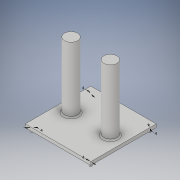
# Autodesk Inventor part: MainStage
Saved by Autodesk Inventor 2019 (Build 230136000, 136)
## iProperties
Created: 2021-06-23
Part Number: MainStage
Material: Generic
Document SubType Name: Modeling
Designer: 91742
Density: 1 g/cm^3
Appearance: Default
Author: 91742
Autodesk Inventor part; units mm, degrees
ref_plane "YZ Plane" through (0, 0, 0) normal (1, 0, 0) x (0, 1, 0)
ref_plane "XZ Plane" through (0, 0, 0) normal (0, 1, 0) x (-1, 0, 0)
ref_plane "XY Plane" through (0, 0, 0) normal (0, 0, 1) x (1, 0, 0)
sketch "Sketch1" plane through (0, 0, 0) normal (0, 1, 0) x (-1, 0, 0)
  line L0 (50, 50) -> (-50, 50)
  line L1 (-50, 50) -> (-50, -50)
  line L2 (-50, -50) -> (50, -50)
  line L3 (50, -50) -> (50, 50)
  line L4 (50, 50) -> (-50, -50) construction
  line L5 (-50, 50) -> (50, -50) construction
  line L6 (-45, 45) -> (45, -45) construction
  line L7 (45, 45) -> (-45, -45) construction
  circle A0 centre (45, -45) radius 2
  circle A1 centre (-45, -45) radius 2
  circle A2 centre (-45, 45) radius 2
  circle A3 centre (45, 45) radius 2
  point P0 (0, 0)
  dimension "d0" = 100
  dimension "d1" = 100
  dimension "d8" = 90
  dimension "d9" = 90
  dimension "d10" = 4
  dimension "d11" = 4
  dimension "d12" = 4
  dimension "d13" = 4
  constraints: 16 end point, 4 centre point, 4 coincident, 3 midpoint, 2 parallel, 1 horizontal, 1 perpendicular
  measures "d0" distance of L2.end L1.end
  measures "d1" distance of L1.end L0.end
  measures "d8" distance of L6.end L7.end
  measures "d9" distance of L7.start L6.end
  measures "d10" diameter of A0
  measures "d11" diameter of A1
  measures "d12" diameter of A2
  measures "d13" diameter of A3
extrude "Extrusion1" add sketch "Sketch1" along normal blind 5
sketch "Sketch2" plane through (0, 0, 0) normal (0, -1, 0) x (1, 0, 0)
  circle A0 centre (45, 45) radius 2
  circle A1 centre (-45, 45) radius 2
  circle A2 centre (-45, -45) radius 2
  circle A3 centre (45, -45) radius 2
  point P0 (0, 0)
  dimension "d16" = 4
  dimension "d17" = 4
  dimension "d18" = 4
  dimension "d19" = 4
  constraints: 4 centre point
  measures "d16" diameter of A0
  measures "d17" diameter of A1
  measures "d18" diameter of A2
  measures "d19" diameter of A3
extrude "Extrusion2" add sketch "Sketch2" along normal mid plane 10
sketch "Sketch5" plane through (0, 5, 0) normal (0, 1, 0) x (1, 0, 0)
  circle A0 centre (-30, 0) radius 10
  circle A1 centre (30, 0) radius 10
  point P0 (0, 0)
  dimension "d36" = 20
  dimension "d37" = 20
  constraints: 2 centre point
  measures "d36" diameter of A0
  measures "d37" diameter of A1
extrude "Extrusion4" add sketch "Sketch5" along normal blind 100
fillet "Fillet1" radius 2 2 edges at (20, 5, 0) (-40, 5, 0)
body "Solid1"
